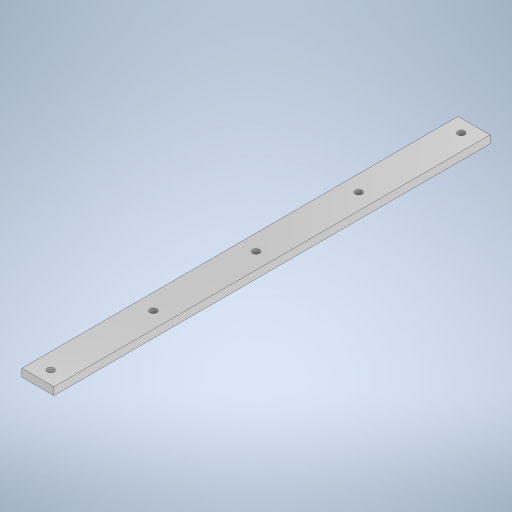
# Autodesk Inventor part: slider_rail_gaba
Saved by Autodesk Inventor 2023 (Build 270158000, 158)
## iProperties
Created: 2021-10-23
Part Number: slider_rail_gaba
Material: アルミニウム 6061-AHC
Document SubType Name: Modeling
Designer: sky
Density: 2.7 g/cm^3
Appearance: アルミニウム - ダーク
Author: sky
Autodesk Inventor part; units mm, degrees
ref_plane "YZ Plane" through (0, 0, 0) normal (1, 0, 0) x (0, 1, 0)
ref_plane "XZ Plane" through (0, 0, 0) normal (0, 1, 0) x (-1, 0, 0)
ref_plane "XY Plane" through (0, 0, 0) normal (0, 0, 1) x (1, 0, 0)
sketch "スケッチ1" plane through (0, 0, 0) normal (0, 1, 0) x (-1, 0, 0)
  line L0 (0, 0) -> (25, 0)
  line L1 (25, 0) -> (25, -340)
  line L2 (25, -340) -> (0, -340)
  line L3 (0, -340) -> (0, 0)
  dimension "d0" = 25
  dimension "d1" = 340
  constraints: 8 end point, 2 parallel, 1 horizontal, 1 perpendicular
  measures "d0" distance of L1.end L2.end
  measures "d1" distance of L0.end L1.end
extrude "押し出し1" add sketch "スケッチ1" along normal blind 6
sketch "スケッチ2" plane through (0, 6, 0) normal (0, 1, 0) x (1, 0, 0)
  line L0 (-25, 0) -> (0, 0) projected
  line L1 (-12.5, 0) -> (-12.5, 340) construction
  line L2 (0, 340) -> (-25, 340) projected
  point P0 (-12.5, 10)
  point P1 (-12.5, 90)
  point P2 (-12.5, 170)
  point P3 (-12.5, 250)
  point P4 (-12.5, 330)
  dimension "d4" = 10
  dimension "d5" = 80
  dimension "d6" = 80
  dimension "d7" = 80
  dimension "d8" = 80
  constraints: 4 point on line, 3 midpoint, 2 end point
  measures "d4" distance from line of point (-12.5, 10) L0
  measures "d5" distance of point (-12.5, 90) point (-12.5, 10)
  measures "d6" distance of point (-12.5, 170) point (-12.5, 90)
  measures "d7" distance of point (-12.5, 250) point (-12.5, 170)
  measures "d8" distance of point (-12.5, 330) point (-12.5, 250)
hole "穴1" at (-12.5, 6, -10) at (-12.5, 6, -90) at (-12.5, 6, -170) at (-12.5, 6, -250) at (-12.5, 6, -330) direction (0, -1, 0) diameter 5.2 depth 30 tip angle 118
sketch "スケッチ3" plane through (0, 0, -340) normal (0, 0, -1) x (-1, 0, 0)
  line L0 (25, 0) -> (25, 6) projected
  line L1 (0, 0) -> (25, 0)
  line L2 (25, 0) -> (25, 6)
  line L3 (25, 6) -> (0, 6)
  line L4 (0, 6) -> (0, 0)
  constraints: 8 end point, 2 parallel, 1 horizontal, 1 perpendicular
sketch "スケッチ5" plane through (-25, 0, 0) normal (0, 0, 1) x (1, 0, 0)
  line L0 (25, 0) -> (0, 0) projected
  line L1 (25, 6) -> (0, 6) projected
  line L2 (0, 0) -> (25, 0)
  line L3 (25, 0) -> (25, 6)
  line L4 (25, 6) -> (0, 6)
  line L5 (0, 6) -> (0, 0)
  constraints: 8 end point, 2 parallel, 1 horizontal, 1 perpendicular
extrude "押し出し3" add sketch "スケッチ5" along normal blind 80
sketch "スケッチ6" plane through (0, 6, 0) normal (0, 1, 0) x (1, 0, 0)
  line L0 (0, 340) -> (0, -80) projected
  circle A0 centre (-12.5, 10) radius 2.6 projected
  point P0 (0, 0)
  point P1 (-12.5, -70)
  dimension "d20" = 12.5
  dimension "d21" = 80
  measures "d20" distance from line of L0 point (-12.5, -70)
  measures "d21" distance of point (-12.5, -70) A0.centre
hole "穴2" at (-12.5, 6, 70) direction (0, -1, 0) diameter 5.2 end through all
sketch "スケッチ7" plane through (0, 0, -340) normal (0, 0, -1) x (-1, 0, 0)
  line L0 (0, 6) -> (25, 6) projected
  line L1 (0, 0) -> (25, 0) projected
  line L2 (25, 6) -> (0, 6)
  line L3 (0, 6) -> (0, 0)
  line L4 (0, 0) -> (25, 0)
  line L5 (25, 0) -> (25, 6)
  constraints: 8 end point, 2 parallel, 1 horizontal, 1 perpendicular
extrude "押し出し4" cut sketch "スケッチ3" against normal blind 80
